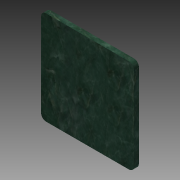
# Autodesk Inventor part: print
Saved by Autodesk Inventor 2015 (Build 190159000, 159)
## iProperties
Created: 2016-01-03
Part Number: print
Material: Generic
Document SubType Name: Modeling
Designer: david
Density: 1 g/cm^3
Appearance: Green Polished
Author: david
Autodesk Inventor part; units mm, degrees
ref_plane "YZ Plane" through (0, 0, 0) normal (1, 0, 0) x (0, 1, 0)
ref_plane "XZ Plane" through (0, 0, 0) normal (0, 1, 0) x (-1, 0, 0)
ref_plane "XY Plane" through (0, 0, 0) normal (0, 0, 1) x (1, 0, 0)
sketch "Sketch1" plane through (0, 0, 0) normal (0, 1, 0) x (-1, 0, 0)
  line L0 (29.5, 28.25) -> (-29.5, 28.25)
  line L1 (-32.5, 25.25) -> (-32.5, -25.25)
  line L2 (-29.5, -28.25) -> (29.5, -28.25)
  line L3 (32.5, -25.25) -> (32.5, 25.25)
  line L4 (32.5, 28.25) -> (-32.5, -28.25) construction
  line L5 (-32.5, 28.25) -> (32.5, -28.25) construction
  arc A0 (32.5, 25.25) -> (29.5, 28.25) centre (29.5, 25.25) ccw
  arc A1 (29.5, -28.25) -> (32.5, -25.25) centre (29.5, -25.25) ccw
  arc A2 (-32.5, -25.25) -> (-29.5, -28.25) centre (-29.5, -25.25) ccw
  arc A3 (-29.5, 28.25) -> (-32.5, 25.25) centre (-29.5, 25.25) ccw
  point P0 (0, 0)
  dimension "d0" = 65
  dimension "d1" = 56.5
  dimension "d2" = 3
  constraints: 12 end point, 8 point on circle, 8 point on line, 8 tangent, 4 centre point, 3 equal radius, 2 midpoint, 2 parallel, 1 horizontal, 1 perpendicular
  measures "d0" distance of L5.end L4.end
  measures "d1" distance of L4.end L5.start
  measures "d2" radius of A0
extrude "Extrusion1" add sketch "Sketch1" along normal blind 3
sketch "Sketch2" plane through (0, 0, 0) normal (0, -1, 0) x (1, 0, 0)
  circle A0 centre (-29, 24.75) radius 1.375
  circle A1 centre (29, 24.75) radius 1.375
  circle A2 centre (29, -24.25) radius 1.375
  circle A3 centre (-29, -24.25) radius 1.375
  line L0 (-32.5, 25.25) -> (-32.5, -25.25) projected
  line L1 (29.5, 28.25) -> (-29.5, 28.25) projected
  point P0 (0, 0)
  dimension "d5" = 2.75
  dimension "d6" = 2.75
  dimension "d7" = 2.75
  dimension "d8" = 2.75
  dimension "d9" = 49
  dimension "d10" = 58
  dimension "d11" = 3.5
  dimension "d12" = 3.5
  dimension "d13" = 3.5
  dimension "d14" = 3.5
  dimension "d15" = 58
  dimension "d16" = 49
  constraints: 4 centre point
  measures "d5" diameter of A0
  measures "d6" diameter of A1
  measures "d7" diameter of A2
  measures "d8" diameter of A3
  measures "d9" distance of A3.centre A0.centre
  measures "d10" distance of A1.centre A0.centre
  measures "d11" distance from line of L0 A0.centre
  measures "d12" distance from line of L1 A0.centre
  measures "d13" distance from line of L1 A1.centre
  measures "d14" distance from line of L0 A3.centre
  measures "d15" distance of A3.centre A2.centre
  measures "d16" distance of A1.centre A2.centre
extrude "Extrusion2" cut sketch "Sketch2" against normal blind 3
body "Solid1"
